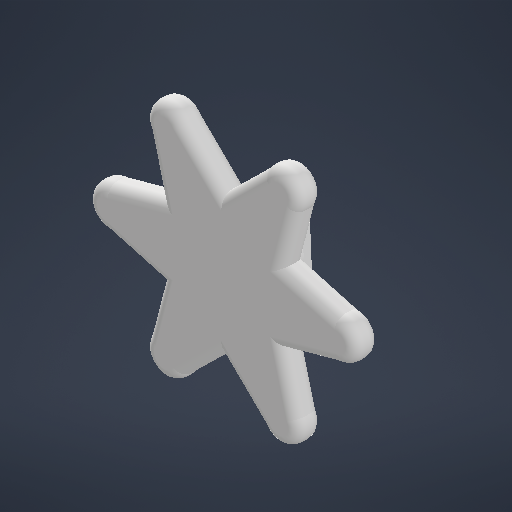
# Autodesk Inventor part: main axel
Saved by Autodesk Inventor 2026 (Build 300175050, 175E)
## iProperties
Created: 2026-04-07
Part Number: main axel
Material: Generic
Document SubType Name: Modeling
Designer: sniel
Density: 1 g/cm^3
Appearance: Default
Author: sniel
Autodesk Inventor part; units mm, degrees
ref_plane "YZ Plane" through (0, 0, 0) normal (1, 0, 0) x (0, 1, 0)
ref_plane "XZ Plane" through (0, 0, 0) normal (0, 1, 0) x (-1, 0, 0)
ref_plane "XY Plane" through (0, 0, 0) normal (0, 0, 1) x (1, 0, 0)
sketch "Sketch1" plane through (0, 0, 0) normal (0, 0, 1) x (1, 0, 0)
  line L0 (4.2481, -3.8751) -> (-3.8751, -4.2481) projected
  line L1 (3.8751, 4.2481) -> (4.2481, -3.8751) projected
  line L2 (-4.2481, 3.8751) -> (3.8751, 4.2481) projected
  line L3 (-3.8751, -4.2481) -> (-4.2481, 3.8751) projected
  arc A0 (-0.3054, 6.0062) -> (0.3054, -6.0062) centre (0, 0) ccw projected
  circle A1 centre (0, 0) radius 5.75
  point P0 (0, 0)
  constraints: 1 coincident, 3 other
extrude "Extrusion1" add sketch "Sketch1" along normal blind 3 contours L0 L3 L2 L1
sketch "Sketch2" plane through (0, 0, 3) normal (0, 0, 1) x (1, 0, 0)
  arc A0 (-0.3054, 6.0062) -> (0.3054, -6.0062) centre (0, 0) ccw
  line L0 (-3.8751, -4.2481) -> (4.2481, -3.8751) projected
  circle A1 centre (0, 0) radius 5.75
  point P0 (0, 0)
  constraints: 2 point on circle, 1 centre point, 1 coincident, 3 other
extrude "Extrusion2" add sketch "Sketch2" along normal blind 6
sketch "Sketch3" plane through (0, 0, 9) normal (0, 0, 1) x (1, 0, 0)
  circle A0 centre (23, 0) radius 4
  circle A1 centre (0, 0) radius 10
  line L0 (23, 4) -> (2.6719, 9.6364)
  line L1 (23, -4) -> (2.6719, -9.6364)
  circle A2 centre (11.5, 19.9186) radius 4
  line L2 (8.0359, 21.9186) -> (-7.0094, 7.1322)
  line L3 (14.9641, 17.9186) -> (9.6814, -2.5043)
  circle A3 centre (-11.5, 19.9186) radius 4
  line L4 (-14.9641, 17.9186) -> (-9.6814, -2.5043)
  line L5 (-8.0359, 21.9186) -> (7.0094, 7.1322)
  circle A4 centre (-23, 0) radius 4
  line L6 (-23, -4) -> (-2.6719, -9.6364)
  line L7 (-23, 4) -> (-2.6719, 9.6364)
  circle A5 centre (-11.5, -19.9186) radius 4
  line L8 (-8.0359, -21.9186) -> (7.0094, -7.1322)
  line L9 (-14.9641, -17.9186) -> (-9.6814, 2.5043)
  circle A6 centre (11.5, -19.9186) radius 4
  line L10 (14.9641, -17.9186) -> (9.6814, 2.5043)
  line L11 (8.0359, -21.9186) -> (-7.0094, -7.1322)
  point P0 (0, 14.021)
  point P1 (-12.1425, 7.0105)
  point P2 (-12.1425, -7.0105)
  point P3 (0, -14.021)
  point P4 (12.1425, -7.0105)
  point P5 (12.1425, 7.0105)
  dimension "d4" = 20
  dimension "d7" = 360
  constraints: 24 end point, 14 point on circle, 7 centre point, 2 tangent, 1 coincident, 49 other
  measures "d4" diameter of A1
extrude "Extrusion3" add sketch "Sketch3" along normal blind 5
fillet "Fillet1" radius 2 36 edges at (13.5533, 12.4645, 14) (13.5, 23.3827, 14) (4.0179, 17.9698, 14) (-4.0179, 17.9698, 14) (-13.5, 23.3827, 14) (-13.5533, 12.4645, 14) (-17.5713, 5.5052, 14) (-27, 0, 14) (-17.5713, -5.5052, 14) (-13.5533, -12.4645, 14) (-13.5, -23.3827, 14) (-4.0179, -17.9698, 14) (4.0179, -17.9698, 14) (13.5, -23.3827, 14) (13.5533, -12.4645, 14) (17.5713, -5.5052, 14) (27, 0, 14) (17.5713, 5.5052, 14) (-13.5533, -12.4645, 9) (-13.5, -23.3827, 9) (-4.0179, -17.9698, 9) (4.0179, -17.9698, 9) (13.5, -23.3827, 9) (13.5533, -12.4645, 9) (17.5713, -5.5052, 9) (17.5713, 5.5052, 9) (27, 0, 9) (13.5533, 12.4645, 9) (13.5, 23.3827, 9) (-4.0179, 17.9698, 9) (-13.5, 23.3827, 9) (-13.5533, 12.4645, 9) (-17.5713, 5.5052, 9) (-27, 0, 9) (-17.5713, -5.5052, 9) (4.0179, 17.9698, 9)
body "Solid1"
